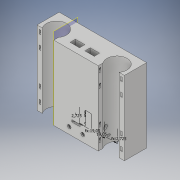
# Autodesk Inventor part: x_carriage
Saved by Autodesk Inventor 2019.4 (Build 234330000, 330)
## iProperties
Created: 2019-07-27
Part Number: x_carriage
Material: Generisch
Document SubType Name: Modeling
Designer: marc
Density: 1 g/cm^3
Appearance: Vorgabe
Author: marc
Autodesk Inventor part; units mm, degrees
sketch "Skizze1" plane through (0, 0, 0) normal (0, 1, 0) x (-1, 0, 0)
  arc A0 (-6, 4.5) -> (6, 4.5) centre (0, 0) ccw
  arc A1 (-51, 4.5) -> (-39, 4.5) centre (-45, 0) ccw
  line L0 (10, -12) -> (-55, -12)
  line L1 (10, -12) -> (10, 4.5)
  line L2 (-6, 4.5) -> (-6, 8)
  line L3 (-6, 8) -> (-39, 8)
  line L4 (-39, 8) -> (-39, 4.5)
  line L5 (-55, -12) -> (-55, 4.5)
  line L6 (-55, 4.5) -> (-51, 4.5)
  line L7 (10, 4.5) -> (6, 4.5)
  dimension "d1" = 15
  dimension "d2" = 15
  dimension "d3" = 45
  dimension "d4" = 65
  dimension "d5" = 10
  dimension "d6" = 10
  dimension "d7" = 12
  dimension "d12" = 6
  dimension "d13" = 6
  dimension "d14" = 8
  constraints: 16 end point, 4 point on circle, 3 horizontal alignment, 3 vertical, 2 centre point, 2 horizontal, 2 perpendicular, 1 coincident, 1 point on line
  measures "d1" diameter of A0
  measures "d2" diameter of A1
  measures "d3" distance of point (0, 0) A1.centre
  measures "d4" distance of L0.start L0.end
  measures "d5" horizontal distance of L0.start point (0, 0)
  measures "d6" horizontal distance of L0.end A1.centre
  measures "d7" distance from line of L0 A1.centre
  measures "d12" distance from line of A1.centre L4
  measures "d13" distance from line of point (0, 0) L2
  measures "d14" distance from line of point (0, 0) L3
extrude "Extrusion1" add sketch "Skizze1" along normal blind 55
sketch "Skizze2" plane through (0, 0, 0) normal (0, -1, 0) x (1, 0, 0)
  circle A0 centre (0, 0) radius 8.5
  circle A1 centre (0, 0) radius 9.25
  line L0 (22.5, -21.3811) -> (22.5, 30.3166)
  line L1 (-10, 4.5) -> (-10, -12) projected
  line L2 (55, -12) -> (55, 4.5) projected
  circle A2 centre (45, 0) radius 8.5
  circle A3 centre (45, 0) radius 9.25
  dimension "d17" = 17
  dimension "d18" = 18.5
  dimension "d19" = 32.5
  dimension "d20" = 32.5
  constraints: 4 centre point, 3 coincident, 2 end point, 2 symmetric about line, 1 vertical, 2 other
  measures "d17" diameter of A0
  measures "d18" diameter of A1
  measures "d19" distance between parallel lines of L1 L0
  measures "d20" distance between parallel lines of L2 L0
ref_plane "Arbeitsebene1" through (0, 5, 0) normal (0, -1, 0) x (1, 0, 0)
ref_plane "Arbeitsebene3" through (0, 50, 0) normal (0, -1, 0) x (1, 0, 0)
ref_plane "Arbeitsebene4" through (0, 15, 0) normal (0, -1, 0) x (1, 0, 0)
ref_plane "Arbeitsebene5" through (0, 40, 0) normal (0, -1, 0) x (1, 0, 0)
sketch "Skizze3" plane through (0, 5, 0) normal (0, -1, 0) x (1, 0, 0)
  circle A0 centre (0, 0) radius 8.5
  circle A1 centre (0, 0) radius 9.5
  line L0 (22.5, -21.3811) -> (22.5, 30.3166)
  circle A2 centre (45, 0) radius 9.5
  circle A3 centre (45, 0) radius 8.5
  dimension "d26" = 17
  dimension "d27" = 19
  dimension "d42" = 45
  constraints: 4 centre point, 3 coincident, 2 end point, 2 symmetric about line, 1 vertical, 2 other
  measures "d26" diameter of A0
  measures "d27" diameter of A1
  measures "d42" distance of point (0, 0) A2.centre
sketch "Skizze4" plane through (0, 50, 0) normal (0, -1, 0) x (1, 0, 0)
  circle A0 centre (0, 0) radius 8.5
  circle A1 centre (0, 0) radius 9.5
  line L0 (22.5, -21.3811) -> (22.5, 30.3166)
  circle A2 centre (45, 0) radius 9.5
  circle A3 centre (45, 0) radius 8.5
  dimension "d30" = 17
  dimension "d31" = 19
  dimension "d43" = 45
  constraints: 4 centre point, 3 coincident, 2 end point, 2 symmetric about line, 1 vertical, 2 other
  measures "d30" diameter of A0
  measures "d31" diameter of A1
  measures "d43" distance of point (0, 0) A2.centre
sketch "Skizze5" plane through (0, 15, 0) normal (0, -1, 0) x (1, 0, 0)
  circle A0 centre (0, 0) radius 8.5
  circle A1 centre (0, 0) radius 9.5
  line L0 (22.5, -21.3811) -> (22.5, 30.3166)
  circle A2 centre (45, 0) radius 9.5
  circle A3 centre (45, 0) radius 8.5
  dimension "d34" = 17
  dimension "d35" = 19
  dimension "d45" = 45
  constraints: 4 centre point, 3 coincident, 2 end point, 2 symmetric about line, 1 vertical, 2 other
  measures "d34" diameter of A0
  measures "d35" diameter of A1
  measures "d45" distance of A2.centre point (0, 0)
sketch "Skizze6" plane through (0, 40, 0) normal (0, -1, 0) x (1, 0, 0)
  circle A0 centre (0, 0) radius 8.5
  circle A1 centre (0, 0) radius 9.5
  line L0 (22.5, -21.3811) -> (22.5, 30.3166)
  circle A2 centre (45, 0) radius 9.5
  circle A3 centre (45, 0) radius 8.5
  dimension "d38" = 17
  dimension "d39" = 19
  dimension "d44" = 45
  constraints: 4 centre point, 3 coincident, 2 end point, 2 symmetric about line, 1 vertical, 2 other
  measures "d38" diameter of A0
  measures "d39" diameter of A1
  measures "d44" distance of A2.centre point (0, 0)
extrude "Extrusion2" cut sketch "Skizze3" against normal blind 3
extrude "Extrusion3" cut sketch "Skizze5" against normal blind 3
extrude "Extrusion4" cut sketch "Skizze6" against normal blind 3
extrude "Extrusion5" cut sketch "Skizze4" against normal blind 3
sketch "Skizze9" plane through (55, 0, -12) normal (0, 0, -1) x (-1, 0, 0)
  line L0 (49.25, 0) -> (15.75, 0)
  line L1 (15.75, 0) -> (15.75, 10.5)
  line L2 (15.75, 10.5) -> (49.25, 10.5)
  line L3 (49.25, 10.5) -> (49.25, 0)
  line L4 (65, 0) -> (0, 0) projected
  line L5 (0, 0) -> (0, 55) projected
  point P0 (55, 0)
  dimension "d74" = 33.5
  dimension "d75" = 10.5
  dimension "d76" = 15.75
  dimension "d77" = 65
  constraints: 8 end point, 2 parallel, 1 horizontal, 1 perpendicular, 1 point on line
  measures "d74" distance of L1.end L2.end
  measures "d75" distance of L0.end L1.end
  measures "d76" distance between parallel lines of L5 L1
  measures "d77" distance of L4.start L4.end
extrude "Extrusion7" cut sketch "Skizze9" against normal blind 3.5
sketch "Skizze11" plane through (55, 0, -8.5) normal (0, 0, -1) x (-1, 0, 0)
  line L0 (49.25, 10.5) -> (49.25, 0) projected
  line L1 (15.75, 0) -> (15.75, 10.5) projected
  line L2 (49.25, 0) -> (15.75, 0) projected
  point P0 (55, 0)
  point P1 (46.525, 5)
  point P2 (37.525, 5)
  point P3 (18.475, 5)
  point P4 (27.475, 5)
  dimension "d81" = 19.05
  dimension "d82" = 19.05
  dimension "d83" = 2.725
  dimension "d84" = 2.725
  dimension "d85" = 5
  constraints: 3 horizontal alignment
  measures "d81" distance of point (18.475, 5) point (37.525, 5)
  measures "d82" distance of point (27.475, 5) point (46.525, 5)
  measures "d83" distance from line of L0 point (46.525, 5)
  measures "d84" distance from line of L1 point (18.475, 5)
  measures "d85" distance from line of L2 point (37.525, 5)
hole "Bohrung1" at (36.525, 5, -8.5) at (8.475, 5, -8.5) direction (0, 0, 1) diameter 2.7 depth 8
sketch "Skizze12" plane through (55, 0, -8.5) normal (0, 0, -1) x (-1, 0, 0)
  line L0 (35.5, 9) -> (29.5, 9)
  line L1 (29.5, 9) -> (29.5, 10.5)
  line L2 (29.5, 10.5) -> (35.5, 10.5)
  line L3 (35.5, 10.5) -> (35.5, 9)
  line L4 (15.75, 0) -> (15.75, 10.5) projected
  line L5 (49.25, 10.5) -> (49.25, 0) projected
  line L6 (15.75, 10.5) -> (49.25, 10.5) projected
  point P0 (55, 0)
  dimension "d93" = 1.5
  dimension "d94" = 6
  dimension "d95" = 13.75
  dimension "d96" = 13.75
  constraints: 8 end point, 2 parallel, 1 horizontal, 1 perpendicular, 1 point on line
  measures "d93" distance of L0.end L1.end
  measures "d94" distance of L0.start L0.end
  measures "d95" distance between parallel lines of L4 L1
  measures "d96" distance between parallel lines of L5 L3
extrude "Extrusion8" cut sketch "Skizze12" against normal up to surface (16.5 mm away)
sketch "Skizze13" plane through (55, 0, -8.5) normal (0, 0, -1) x (-1, 0, 0)
  circle A0 centre (46.525, 5) radius 1.35 projected
  circle A1 centre (18.475, 5) radius 1.35 projected
  line L0 (49.25, 0) -> (15.75, 0) projected
  line L1 (15.75, 0) -> (15.75, 10.5) projected
  line L2 (15.75, 10.5) -> (29.5, 10.5) projected
  line L3 (35.5, 9) -> (29.5, 9) projected
  line L4 (29.5, 9) -> (29.5, 10.5) projected
  line L5 (35.5, 10.5) -> (35.5, 9) projected
  line L6 (35.5, 10.5) -> (49.25, 10.5) projected
  line L7 (49.25, 10.5) -> (49.25, 0) projected
  circle A2 centre (46.525, 5) radius 2
  circle A3 centre (37.525, 5) radius 2
  circle A4 centre (27.475, 5) radius 2
  circle A5 centre (18.475, 5) radius 2
  point P0 (55, 0)
  dimension "d99" = 4
  dimension "d100" = 4
  dimension "d101" = 4
  dimension "d102" = 4
  constraints: 4 centre point, 4 coincident
  measures "d99" diameter of A2
  measures "d100" diameter of A3
  measures "d101" diameter of A4
  measures "d102" diameter of A5
extrude "Extrusion9" cut sketch "Skizze13" against normal blind 0.75 contours L0 L1 L2 L4 L3 L5 L6 L7
sketch "Skizze14" plane through (0, 0, 0) normal (0, -1, 0) x (1, 0, 0)
  point P0 (0, 0)
sketch "Skizze15" plane through (0, 0, 0) normal (0, -1, 0) x (1, 0, 0)
  line L0 (13.5, -0.6) -> (20.5, -0.6)
  line L1 (20.5, -0.6) -> (20.5, 3.4)
  line L2 (20.5, 3.4) -> (13.5, 3.4)
  line L3 (13.5, 3.4) -> (13.5, -0.6)
  line L4 (39.25, -12) -> (5.75, -12) projected
  line L5 (24.5, -0.6) -> (31.5, -0.6)
  line L6 (31.5, -0.6) -> (31.5, 3.4)
  line L7 (31.5, 3.4) -> (24.5, 3.4)
  line L8 (24.5, 3.4) -> (24.5, -0.6)
  point P0 (0, 0)
  dimension "d105" = 13.5
  dimension "d106" = 11.4
  dimension "d107" = 7
  dimension "d108" = 4
  dimension "d109" = 7
  dimension "d110" = 4
  dimension "d111" = 4
  constraints: 16 end point, 4 parallel, 2 horizontal, 2 perpendicular, 1 collinear
  measures "d105" distance from line of point (0, 0) L3
  measures "d106" distance between parallel lines of L4 L0
  measures "d107" distance of L0.start L0.end
  measures "d108" distance of L0.end L1.end
  measures "d109" distance of L7.end L6.end
  measures "d110" distance of L6.end L5.end
  measures "d111" distance between parallel lines of L1 L8
extrude "Extrusion10" cut sketch "Skizze15" against normal up to surface (55 mm away)
hole "Bohrung2" at (17.475, 5, -8.5) at (27.525, 5, -8.5) direction (0, 0, 1) diameter 2.7 end through all
sketch "Skizze16" plane through (0, 0, 0) normal (0, -1, 0) x (1, 0, 0)
  line L0 (31.5, 3.4) -> (31.5, -0.6) projected
  line L1 (31.5, 2.9) -> (32, 2.9)
  line L2 (32, 2.9) -> (32, 4.9)
  line L3 (32, 4.9) -> (31.5, 4.9)
  line L4 (31.5, 4.9) -> (31.5, 2.9)
  line L5 (24.5, 2.9) -> (24, 2.9)
  line L6 (24, 2.9) -> (24, 4.9)
  line L7 (24, 4.9) -> (24.5, 4.9)
  line L8 (24.5, 4.9) -> (24.5, 2.9)
  line L9 (20.5, 3.4) -> (20.5, -0.6) projected
  line L10 (20.5, 2.9) -> (21, 2.9)
  line L11 (21, 2.9) -> (21, 4.9)
  line L12 (21, 4.9) -> (20.5, 4.9)
  line L13 (20.5, 4.9) -> (20.5, 2.9)
  line L14 (13.5, 2.9) -> (13, 2.9)
  line L15 (13, 2.9) -> (13, 4.9)
  line L16 (13, 4.9) -> (13.5, 4.9)
  line L17 (13.5, 4.9) -> (13.5, 2.9)
  line L18 (24.5, -0.6) -> (24.5, 3.4) projected
  line L19 (24.5, 3.4) -> (31.5, 3.4) projected
  line L20 (13.5, -0.6) -> (13.5, 3.4) projected
  line L21 (32, 4.9) -> (24, 4.9)
  line L22 (24, 4.9) -> (24, 5.1)
  line L23 (24, 5.1) -> (32, 5.1)
  line L24 (32, 5.1) -> (32, 4.9)
  line L25 (21, 4.9) -> (13, 4.9)
  line L26 (13, 4.9) -> (13, 5.1)
  line L27 (13, 5.1) -> (21, 5.1)
  line L28 (21, 5.1) -> (21, 4.9)
  point P0 (0, 0)
  dimension "d121" = 0.5
  dimension "d122" = 0.5
  dimension "d123" = 0.5
  dimension "d124" = 0.5
  dimension "d125" = 0.5
  dimension "d126" = 1.5
  dimension "d127" = 0.2
  dimension "d128" = 0.2
  constraints: 48 end point, 12 parallel, 10 point on line, 6 horizontal, 6 perpendicular
  measures "d121" distance between parallel lines of L13 L11
  measures "d122" distance between parallel lines of L8 L6
  measures "d123" distance between parallel lines of L2 L4
  measures "d124" distance between parallel lines of L17 L15
  measures "d125" distance between parallel lines of L19 L5
  measures "d126" distance between parallel lines of L19 L7
  measures "d127" distance between parallel lines of L21 L23
  measures "d128" distance between parallel lines of L25 L27
extrude "Extrusion11" [suppressed]
sketch "Skizze17" plane through (31.5, 55, 3.4) normal (0, 0, -1) x (-1, 0, 0)
  circle A0 centre (3.975, -50) radius 1.35 projected
  circle A1 centre (14.025, -50) radius 1.35 projected
  point P0 (31.5, -55)
extrude "Extrusion12" [suppressed]
sketch "Skizze18" plane through (24.5, 0, -0.6) normal (0, 0, 1) x (1, 0, 0)
  circle A0 centre (3.025, 5) radius 1.35 projected
  circle A1 centre (-7.025, 5) radius 1.35 projected
  point P0 (-24.5, 0)
extrude "Extrusion13" [suppressed]
ref_plane "Arbeitsebene6" through (3, 0, -12) normal (-1, 0, 0) x (0, 0, 1)
sketch "Skizze19" plane through (3, 0, -12) normal (-1, 0, 0) x (0, 0, 1)
  line L0 (20, 0) -> (16.5, 0) projected
  point P0 (12, 0)
  point P1 (13.4, 11.5)
  point P2 (0, 0)
  dimension "d136" = 13.4
  dimension "d137" = 11.5
  measures "d136" horizontal distance of point (0, 0) point (13.4, 11.5)
  measures "d137" distance from line of L0 point (13.4, 11.5)
hole "Bohrung3" at (3, 11.5, 1.4) direction (1, 0, 0) diameter 3.4 depth 38.75 counterbore diameter 8 counterbore depth 6.5
sketch "Skizze20" plane through (0, 0, 0) normal (0, -1, 0) x (1, 0, 0)
  line L0 (14.675, 4.75) -> (20.275, 4.75)
  line L1 (20.275, 4.75) -> (20.275, 7.25)
  line L2 (20.275, 7.25) -> (14.675, 7.25)
  line L3 (14.675, 7.25) -> (14.675, 4.75)
  line L4 (14.675, 4.75) -> (20.275, 7.25) construction
  line L5 (20.275, 4.75) -> (14.675, 7.25) construction
  line L6 (16.125, 8) -> (18.825, 8) projected
  line L7 (39.25, -7.75) -> (39.25, -12) projected
  line L8 (39, 8) -> (6, 8) projected
  line L9 (24.725, 4.75) -> (30.325, 4.75)
  line L10 (30.325, 4.75) -> (30.325, 7.25)
  line L11 (30.325, 7.25) -> (24.725, 7.25)
  line L12 (24.725, 7.25) -> (24.725, 4.75)
  line L13 (24.725, 4.75) -> (30.325, 7.25) construction
  line L14 (30.325, 4.75) -> (24.725, 7.25) construction
  line L15 (5.75, -12) -> (5.75, -7.75) projected
  point P0 (0, 0)
  point P1 (17.475, 6)
  point P2 (27.525, 6)
  dimension "d145" = 5.6
  dimension "d146" = 2.5
  dimension "d147" = 21.775
  dimension "d148" = 2
  dimension "d149" = 5.6
  dimension "d150" = 2.5
  dimension "d151" = 21.775
  dimension "d152" = 2
  constraints: 24 end point, 4 midpoint, 4 parallel, 2 horizontal, 2 perpendicular
  measures "d145" distance of L2.end L1.end
  measures "d146" distance of L1.end L0.end
  measures "d147" distance from line of L7 point (17.475, 6)
  measures "d148" distance from line of L8 point (17.475, 6)
  measures "d149" distance of L10.end L11.end
  measures "d150" distance of L11.end L9.start
  measures "d151" distance from line of L15 point (27.525, 6)
  measures "d152" distance from line of L8 point (27.525, 6)
extrude "Extrusion14" cut sketch "Skizze20" against normal blind 10
equation "\"d2\" = d1"
equation "\"d13\" = d12"
equation "\"d76\" = -0.5 * d74 + 0.5 * d77"
equation "\"d82\" = d81"
equation "\"d84\" = d83"
equation "\"d110\" = d108"
equation "\"d122\" = d121"
equation "\"d123\" = d122"
equation "\"d124\" = d121"
equation "\"d128\" = d127"
equation "\"d147\" = d84 + d81"
equation "\"d149\" = d145"
equation "\"d150\" = d146"
equation "\"d151\" = d147"
equation "\"d152\" = d148"
